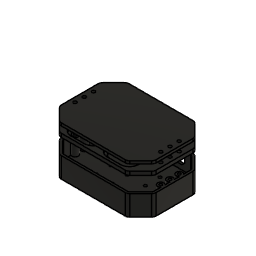
main (Autodesk Fusion 360 design; units mm, degrees)
Autodesk Fusion 360 part; units mm, degrees
sketch "main" plane through (0, 0, 16) normal (0, 0, 1) x (-1, 0, 0)
  line L0 (-15.9568, -31.9728) -> (-28.9568, -28.4593)
  arc A0 (-34.5, -21.219) -> (-28.9568, -28.4593) centre (-27, -21.219) ccw
  line L1 (-34.5, -21.219) -> (-34.5, 21.219)
  arc A1 (-28.9568, 28.4593) -> (-34.5, 21.219) centre (-27, 21.219) ccw
  line L2 (-28.9568, 28.4593) -> (-15.9568, 31.9728)
  arc A2 (-6.5, 24.7326) -> (-15.9568, 31.9728) centre (-14, 24.7326) ccw
  line L3 (-6.5, 24.7326) -> (-6.5, -24.7326)
  arc A3 (-15.9568, -31.9728) -> (-6.5, -24.7326) centre (-14, -24.7326) ccw
  line L4 (-7.8009, -43.5) -> (0, -43.5)
  line L5 (0, -43.5) -> (7.8009, -43.5)
  line L6 (7.8009, -43.5) -> (40.1741, -34.7505)
  arc A4 (40.1741, -34.7505) -> (43.5, -30.4063) centre (39, -30.4063) ccw
  line L7 (43.5, -30.4063) -> (43.5, 30.4063)
  arc A5 (43.5, 30.4063) -> (40.1741, 34.7505) centre (39, 30.4063) ccw
  line L8 (40.1741, 34.7505) -> (7.8009, 43.5)
  line L9 (7.8009, 43.5) -> (-7.8009, 43.5)
  line L10 (-7.8009, 43.5) -> (-40.1741, 34.7505)
  arc A6 (-40.1741, 34.7505) -> (-43.5, 30.4063) centre (-39, 30.4063) ccw
  line L11 (-43.5, 30.4063) -> (-43.5, -30.4063)
  arc A7 (-43.5, -30.4063) -> (-40.1741, -34.7505) centre (-39, -30.4063) ccw
  line L12 (-40.1741, -34.7505) -> (-7.8009, -43.5)
  arc A8 (6.5, -24.7326) -> (15.9568, -31.9728) centre (14, -24.7326) ccw
  line L13 (6.5, -24.7326) -> (6.5, 24.7326)
  arc A9 (15.9568, 31.9728) -> (6.5, 24.7326) centre (14, 24.7326) ccw
  line L14 (15.9568, 31.9728) -> (28.9568, 28.4593)
  arc A10 (34.5, 21.219) -> (28.9568, 28.4593) centre (27, 21.219) ccw
  line L15 (34.5, 21.219) -> (34.5, -21.219)
  arc A11 (28.9568, -28.4593) -> (34.5, -21.219) centre (27, -21.219) ccw
  line L16 (28.9568, -28.4593) -> (15.9568, -31.9728)
  line L17 (37, 34.5) -> (-37, 34.5) construction
  line L18 (-37, 34.5) -> (-37, -34.5) construction
  line L19 (-37, -34.5) -> (37, -34.5) construction
  line L20 (37, -34.5) -> (37, 34.5) construction
  line L21 (37, 34.5) -> (-37, -34.5) construction
  line L22 (-37, 34.5) -> (37, -34.5) construction
  line L23 (-37, -34.5) -> (-3, -34.5) construction
  line L24 (-3, -34.5) -> (-3, -0.5) construction
  line L25 (-3, -0.5) -> (-37, -0.5) construction
  line L26 (-37, -0.5) -> (-37, -34.5) construction
  line L27 (-37, 34.5) -> (-3, 34.5) construction
  line L28 (-3, 34.5) -> (-3, 0.5) construction
  line L29 (-3, 0.5) -> (-37, 0.5) construction
  line L30 (-37, 0.5) -> (-37, 34.5) construction
  line L31 (37, 34.5) -> (3, 34.5) construction
  line L32 (3, 34.5) -> (3, 0.5) construction
  line L33 (3, 0.5) -> (37, 0.5) construction
  line L34 (37, 0.5) -> (37, 34.5) construction
  line L35 (37, -34.5) -> (3, -34.5) construction
  line L36 (3, -34.5) -> (3, -0.5) construction
  line L37 (3, -0.5) -> (37, -0.5) construction
  line L38 (37, -0.5) -> (37, -34.5) construction
  line L39 (-37, -0.5) -> (-3, -34.5) construction
  line L40 (-3, -0.5) -> (-37, -34.5) construction
  line L41 (-37, 34.5) -> (-3, 0.5) construction
  line L42 (-3, 34.5) -> (-37, 0.5) construction
  line L43 (3, 34.5) -> (37, 0.5) construction
  line L44 (37, 34.5) -> (3, 0.5) construction
  line L45 (3, -34.5) -> (37, -0.5) construction
  line L46 (37, -34.5) -> (3, -0.5) construction
  line L47 (-12.7, -0.2) -> (-27.3, -0.2)
  line L48 (-37.3, -10.2) -> (-37.3, -24.8)
  line L49 (-27.3, -34.8) -> (-12.7, -34.8)
  line L50 (-2.7, -24.8) -> (-2.7, -10.2)
  line L51 (-2.7, -0.2) -> (-37.3, -34.8) construction
  line L52 (-37.3, -0.2) -> (-2.7, -34.8) construction
  line L53 (-12.7, 34.8) -> (-27.3, 34.8)
  line L54 (-37.3, 24.8) -> (-37.3, 10.2)
  line L55 (-27.3, 0.2) -> (-12.7, 0.2)
  line L56 (-2.7, 10.2) -> (-2.7, 24.8)
  line L57 (-2.7, 34.8) -> (-37.3, 0.2) construction
  line L58 (-37.3, 34.8) -> (-2.7, 0.2) construction
  line L59 (27.3, 34.8) -> (12.7, 34.8)
  line L60 (2.7, 24.8) -> (2.7, 10.2)
  line L61 (12.7, 0.2) -> (27.3, 0.2)
  line L62 (37.3, 10.2) -> (37.3, 24.8)
  line L63 (37.3, 34.8) -> (2.7, 0.2) construction
  line L64 (2.7, 34.8) -> (37.3, 0.2) construction
  line L65 (27.3, -0.2) -> (12.7, -0.2)
  line L66 (2.7, -10.2) -> (2.7, -24.8)
  line L67 (12.7, -34.8) -> (27.3, -34.8)
  line L68 (37.3, -24.8) -> (37.3, -10.2)
  line L69 (37.3, -0.2) -> (2.7, -34.8) construction
  line L70 (2.7, -0.2) -> (37.3, -34.8) construction
  arc A12 (-27.3, 34.8) -> (-37.3, 24.8) centre (-27.3, 24.8) ccw
  arc A13 (-37.3, 10.2) -> (-27.3, 0.2) centre (-27.3, 10.2) ccw
  arc A14 (-12.7, 0.2) -> (-2.7, 10.2) centre (-12.7, 10.2) ccw
  arc A15 (-2.7, 24.8) -> (-12.7, 34.8) centre (-12.7, 24.8) ccw
  arc A16 (12.7, 34.8) -> (2.7, 24.8) centre (12.7, 24.8) ccw
  arc A17 (37.3, 24.8) -> (27.3, 34.8) centre (27.3, 24.8) ccw
  arc A18 (27.3, 0.2) -> (37.3, 10.2) centre (27.3, 10.2) ccw
  arc A19 (2.7, 10.2) -> (12.7, 0.2) centre (12.7, 10.2) ccw
  arc A20 (-37.3, -24.8) -> (-27.3, -34.8) centre (-27.3, -24.8) ccw
  arc A21 (-12.7, -34.8) -> (-2.7, -24.8) centre (-12.7, -24.8) ccw
  arc A22 (-2.7, -10.2) -> (-12.7, -0.2) centre (-12.7, -10.2) ccw
  arc A23 (-27.3, -0.2) -> (-37.3, -10.2) centre (-27.3, -10.2) ccw
  arc A24 (12.7, -0.2) -> (2.7, -10.2) centre (12.7, -10.2) ccw
  arc A25 (2.7, -24.8) -> (12.7, -34.8) centre (12.7, -24.8) ccw
  arc A26 (27.3, -34.8) -> (37.3, -24.8) centre (27.3, -24.8) ccw
  arc A27 (37.3, -10.2) -> (27.3, -0.2) centre (27.3, -10.2) ccw
  arc A28 (-34.3, -24.8) -> (-27.3, -31.8) centre (-27.3, -24.8) ccw
  line L71 (-27.3, -31.8) -> (-12.7, -31.8)
  arc A29 (-12.7, -31.8) -> (-5.7, -24.8) centre (-12.7, -24.8) ccw
  line L72 (-5.7, -24.8) -> (-5.7, -10.2)
  arc A30 (-5.7, -10.2) -> (-12.7, -3.2) centre (-12.7, -10.2) ccw
  line L73 (-12.7, -3.2) -> (-27.3, -3.2)
  arc A31 (-27.3, -3.2) -> (-34.3, -10.2) centre (-27.3, -10.2) ccw
  line L74 (-34.3, -10.2) -> (-34.3, -24.8)
  arc A32 (-12.7, 3.2) -> (-5.7, 10.2) centre (-12.7, 10.2) ccw
  line L75 (-5.7, 10.2) -> (-5.7, 24.8)
  arc A33 (-5.7, 24.8) -> (-12.7, 31.8) centre (-12.7, 24.8) ccw
  line L76 (-12.7, 31.8) -> (-27.3, 31.8)
  arc A34 (-27.3, 31.8) -> (-34.3, 24.8) centre (-27.3, 24.8) ccw
  line L77 (-34.3, 24.8) -> (-34.3, 10.2)
  arc A35 (-34.3, 10.2) -> (-27.3, 3.2) centre (-27.3, 10.2) ccw
  line L78 (-27.3, 3.2) -> (-12.7, 3.2)
  line L79 (5.7, 24.8) -> (5.7, 10.2)
  arc A36 (5.7, 10.2) -> (12.7, 3.2) centre (12.7, 10.2) ccw
  line L80 (12.7, 3.2) -> (27.3, 3.2)
  arc A37 (27.3, 3.2) -> (34.3, 10.2) centre (27.3, 10.2) ccw
  line L81 (34.3, 10.2) -> (34.3, 24.8)
  arc A38 (34.3, 24.8) -> (27.3, 31.8) centre (27.3, 24.8) ccw
  line L82 (27.3, 31.8) -> (12.7, 31.8)
  arc A39 (12.7, 31.8) -> (5.7, 24.8) centre (12.7, 24.8) ccw
  arc A40 (12.7, -3.2) -> (5.7, -10.2) centre (12.7, -10.2) ccw
  line L83 (5.7, -10.2) -> (5.7, -24.8)
  arc A41 (5.7, -24.8) -> (12.7, -31.8) centre (12.7, -24.8) ccw
  line L84 (12.7, -31.8) -> (27.3, -31.8)
  arc A42 (27.3, -31.8) -> (34.3, -24.8) centre (27.3, -24.8) ccw
  line L85 (34.3, -24.8) -> (34.3, -10.2)
  arc A43 (34.3, -10.2) -> (27.3, -3.2) centre (27.3, -10.2) ccw
  line L86 (27.3, -3.2) -> (12.7, -3.2)
  line L87 (35.4289, 37.5) -> (-35.4289, 37.5)
  line L88 (-52.5, 20.4289) -> (-52.5, -20.4289)
  line L89 (-35.4289, -37.5) -> (35.4289, -37.5)
  line L90 (52.5, -20.4289) -> (52.5, 20.4289)
  line L91 (52.5, 37.5) -> (-52.5, -37.5) construction
  line L92 (-52.5, 37.5) -> (52.5, -37.5) construction
  line L93 (-38.9645, -36.0355) -> (-51.0355, -23.9645)
  line L94 (-38.9645, 36.0355) -> (-51.0355, 23.9645)
  line L95 (38.9645, 36.0355) -> (51.0355, 23.9645)
  line L96 (38.9645, -36.0355) -> (51.0355, -23.9645)
  arc A44 (-38.9645, -36.0355) -> (-35.4289, -37.5) centre (-35.4289, -32.5) ccw
  arc A45 (-52.5, -20.4289) -> (-51.0355, -23.9645) centre (-47.5, -20.4289) ccw
  arc A46 (-51.0355, 23.9645) -> (-52.5, 20.4289) centre (-47.5, 20.4289) ccw
  arc A47 (-35.4289, 37.5) -> (-38.9645, 36.0355) centre (-35.4289, 32.5) ccw
  arc A48 (38.9645, 36.0355) -> (35.4289, 37.5) centre (35.4289, 32.5) ccw
  arc A49 (52.5, 20.4289) -> (51.0355, 23.9645) centre (47.5, 20.4289) ccw
  arc A50 (51.0355, -23.9645) -> (52.5, -20.4289) centre (47.5, -20.4289) ccw
  arc A51 (35.4289, -37.5) -> (38.9645, -36.0355) centre (35.4289, -32.5) ccw
  line L97 (-52.5, 20.4289) -> (-42.5, 20.4289) construction
  line L98 (-42.5, 20.4289) -> (-42.5, -20.4289) construction
  line L99 (-42.5, -20.4289) -> (-52.5, -20.4289) construction
  line L100 (-52.5, -20.4289) -> (-52.5, 20.4289) construction
  line L101 (-52.5, 20.4289) -> (-42.5, -20.4289) construction
  line L102 (-42.5, 20.4289) -> (-52.5, -20.4289) construction
  circle A52 centre (-47.5, 0) radius 1.8
  line L103 (-52.5, 20.4289) -> (-42.5, 0) construction
  line L104 (-42.5, 20.4289) -> (-52.5, 0) construction
  line L105 (-52.5, -20.4289) -> (-42.5, 0) construction
  line L106 (-42.5, -20.4289) -> (-52.5, 0) construction
  circle A53 centre (-47.5, -10.2145) radius 1.8
  circle A54 centre (-47.5, 10.2145) radius 1.8
  line L107 (52.5, 20.4289) -> (52.5, -20.4289)
  line L108 (52.5, 20.4289) -> (42.5, 20.4289) construction
  line L109 (42.5, 20.4289) -> (42.5, -20.4291) construction
  line L110 (42.5, -20.4291) -> (52.5, -20.4291) construction
  line L111 (52.5, -20.4291) -> (52.5, 20.4289) construction
  line L112 (42.5, 20.4289) -> (52.5, -20.4289) construction
  line L113 (52.5, 20.4289) -> (42.5, -20.4291) construction
  line L114 (42.5, 20.4289) -> (52.5, 0) construction
  line L115 (52.5, 20.4289) -> (42.5, -0.0001) construction
  line L116 (42.5, -0.0001) -> (52.5, -20.4289) construction
  line L117 (52.5, 0) -> (42.5, -20.4291) construction
  circle A55 centre (47.5, 10.2145) radius 1.8
  circle A56 centre (47.5, -0.0001) radius 1.8
  circle A57 centre (47.5, -10.2145) radius 1.8
  point P0 (-20, -17.5)
  point P1 (-20, 17.5)
  point P2 (20, 17.5)
  point P3 (20, -17.5)
  point P4 (-37.5, -37.5)
  point P5 (-52.5, -22.5)
  point P6 (-37.5, 37.5)
  point P7 (-52.5, 22.5)
  point P8 (37.5, 37.5)
  point P9 (52.5, 22.5)
  point P10 (37.5, -37.5)
  point P11 (52.5, -22.5)
  dimension "d3" = 74
  dimension "d4" = 69
  dimension "d5" = 34
  dimension "d6" = 34
  dimension "d7" = 34
  dimension "d8" = 34
  dimension "d9" = 34
  dimension "d10" = 34
  dimension "d11" = 34
  dimension "d12" = 34
  dimension "d13" = 34.6
  dimension "d14" = 34.6
  dimension "d15" = 34.6
  dimension "d16" = 34.6
  dimension "d17" = 34.6
  dimension "d18" = 34.6
  dimension "d19" = 34.6
  dimension "d20" = 34.6
  dimension "d21" = 10
  dimension "d22" = 10
  dimension "d23" = 10
  dimension "d24" = 10
  dimension "d25" = 10
  dimension "d26" = 10
  dimension "d27" = 10
  dimension "d28" = 10
  dimension "d29" = 10
  dimension "d30" = 10
  dimension "d31" = 10
  dimension "d32" = 10
  dimension "d33" = 10
  dimension "d34" = 10
  dimension "d35" = 10
  dimension "d36" = 10
  dimension "d37" = -3
  dimension "d38" = -3
  dimension "d39" = -3
  dimension "d40" = -3
  dimension "d41" = 105
  dimension "d42" = 75
  dimension "d43" = 15
  dimension "d44" = 15
  dimension "d45" = 15
  dimension "d46" = 15
  dimension "d47" = 15
  dimension "d48" = 15
  dimension "d49" = 15
  dimension "d50" = 15
  dimension "d51" = 5
  dimension "d52" = 5
  dimension "d53" = 5
  dimension "d54" = 5
  dimension "d55" = 5
  dimension "d56" = 5
  dimension "d57" = 5
  dimension "d58" = 5
  dimension "d70" = 10
  dimension "d72" = 3.6
  dimension "d74" = 3.6
  dimension "d75" = 3.6
  dimension "d80" = 10
  dimension "d81" = 40.858
  dimension "d82" = 3.6
  dimension "d83" = 3.6
  dimension "d84" = 3.6
  constraint horizontal L17
  constraint perpendicular L17 L18
  constraint parallel L17 L19
  constraint parallel L18 L20
  constraint coincident L21 origin
  constraint coincident L22 origin
  constraint horizontal L23
  constraint vertical L24
  constraint horizontal L25
  constraint vertical L26
  constraint horizontal L27
  constraint vertical L28
  constraint horizontal L29
  constraint vertical L30
  constraint horizontal L31
  constraint vertical L32
  constraint horizontal L33
  constraint vertical L34
  constraint horizontal L35
  constraint vertical L36
  constraint horizontal L37
  constraint vertical L38
  constraint horizontal L47
  constraint perpendicular L47 L48
  constraint parallel L47 L49
  constraint parallel L48 L50
  constraint coincident L51 P0
  constraint coincident L52 P0
  constraint midpoint L39 P0
  constraint horizontal L53
  constraint perpendicular L53 L54
  constraint parallel L53 L55
  constraint parallel L54 L56
  constraint coincident L57 P1
  constraint coincident L58 P1
  constraint midpoint L42 P1
  constraint horizontal L59
  constraint perpendicular L59 L60
  constraint parallel L59 L61
  constraint parallel L60 L62
  constraint coincident L63 P2
  constraint coincident L64 P2
  constraint midpoint L44 P2
  constraint horizontal L65
  constraint perpendicular L65 L66
  constraint parallel L65 L67
  constraint parallel L66 L68
  constraint coincident L69 P3
  constraint coincident L70 P3
  constraint midpoint L46 P3
  constraint coincident L58.start L54
  constraint coincident L58.start L53
  constraint tangent L54 A12
  constraint tangent L53 A12
  constraint coincident L57.end L55
  constraint coincident L57.end L54
  constraint tangent L55 A13
  constraint tangent L54 A13
  constraint coincident L58.end L55
  constraint coincident L58.end L56
  constraint tangent L55 A14
  constraint tangent L56 A14
  constraint coincident L57.start L56
  constraint coincident L57.start L53
  constraint tangent L56 A15
  constraint tangent L53 A15
  constraint coincident L64.start L59
  constraint coincident L64.start L60
  constraint tangent L59 A16
  constraint tangent L60 A16
  constraint coincident L63.start L59
  constraint coincident L63.start L62
  constraint tangent L59 A17
  constraint tangent L62 A17
  constraint coincident L64.end L62
  constraint coincident L64.end L61
  constraint tangent L62 A18
  constraint tangent L61 A18
  constraint coincident L63.end L61
  constraint coincident L63.end L60
  constraint tangent L61 A19
  constraint tangent L60 A19
  constraint coincident L51.end L49
  constraint coincident L51.end L48
  constraint tangent L49 A20
  constraint tangent L48 A20
  constraint coincident L52.end L49
  constraint coincident L52.end L50
  constraint tangent L49 A21
  constraint tangent L50 A21
  constraint coincident L51.start L50
  constraint coincident L51.start L47
  constraint tangent L50 A22
  constraint tangent L47 A22
  constraint coincident L52.start L47
  constraint coincident L52.start L48
  constraint tangent L47 A23
  constraint tangent L48 A23
  constraint coincident L70.start L66
  constraint coincident L70.start L65
  constraint tangent L66 A24
  constraint tangent L65 A24
  constraint coincident L69.end L67
  constraint coincident L69.end L66
  constraint tangent L67 A25
  constraint tangent L66 A25
  constraint coincident L70.end L67
  constraint coincident L70.end L68
  constraint tangent L67 A26
  constraint tangent L68 A26
  constraint coincident L69.start L68
  constraint coincident L69.start L65
  constraint tangent L68 A27
  constraint tangent L65 A27
  constraint horizontal L87
  constraint perpendicular L87 L88
  constraint parallel L87 L89
  constraint parallel L88 L90
  constraint coincident L91 origin
  constraint coincident L92 origin
  constraint coincident L91.end L89
  constraint coincident L91.end L88
  constraint coincident L92.start L87
  constraint coincident L92.start L88
  constraint coincident L91.start L87
  constraint coincident L91.start L90
  constraint coincident L92.end L89
  constraint coincident L92.end L90
  constraint coincident L89 P4
  constraint coincident P4 L93
  constraint tangent L89 A44
  constraint tangent L93 A44
  constraint coincident P5 L93
  constraint coincident L88 P5
  constraint tangent L93 A45
  constraint tangent L88 A45
  constraint coincident P7 L94
  constraint coincident L88 P7
  constraint tangent L94 A46
  constraint tangent L88 A46
  constraint coincident P6 L94
  constraint coincident L87 P6
  constraint tangent L94 A47
  constraint tangent L87 A47
  constraint coincident P8 L95
  constraint coincident L87 P8
  constraint tangent L95 A48
  constraint tangent L87 A48
  constraint coincident P9 L95
  constraint coincident L90 P9
  constraint tangent L95 A49
  constraint tangent L90 A49
  constraint coincident P11 L96
  constraint coincident L90 P11
  constraint tangent L96 A50
  constraint tangent L90 A50
  constraint coincident P10 L96
  constraint coincident L89 P10
  constraint tangent L96 A51
  constraint tangent L89 A51
  constraint horizontal L97
  constraint vertical L98
  constraint horizontal L99
  constraint vertical L100
  constraint midpoint L101 A52.centre
  constraint midpoint L98 L103.end
  constraint midpoint L100 L104.end
  constraint midpoint L106 A53.centre
  constraint midpoint L104 A54.centre
  constraint horizontal L108
  constraint vertical L109
  constraint horizontal L110
  constraint vertical L111
  constraint midpoint L107 L114.end
  constraint midpoint L109 L115.end
  constraint midpoint L114 A55.centre
  constraint midpoint L113 A56.centre
  constraint midpoint L117 A57.centre
  measures "d3" distance of L18.end L19.end
  measures "d4" distance of L17.end L18.end
  measures "d5" distance of L18.end L23.end
  measures "d6" distance of L18.end L25.end
  measures "d7" distance of L17.end L27.end
  measures "d8" distance of L17.end L29.end
  measures "d9" distance of L17.start L31.end
  measures "d10" distance of L17.start L33.end
  measures "d11" distance of L19.end L35.end
  measures "d12" distance of L19.end L37.end
  measures "d13" distance of L51.end L52.end
  measures "d14" distance of L52.start L51.end
  measures "d15" distance of L57.end L58.end
  measures "d16" distance of L58.start L57.end
  measures "d17" distance of L63.end L64.end
  measures "d18" distance of L64.start L63.end
  measures "d19" distance of L69.end L70.end
  measures "d20" distance of L70.start L69.end
  measures "d21" radius of A12
  measures "d22" radius of A13
  measures "d23" radius of A14
  measures "d24" radius of A15
  measures "d25" radius of A16
  measures "d26" radius of A17
  measures "d27" radius of A18
  measures "d28" radius of A19
  measures "d29" radius of A20
  measures "d30" radius of A21
  measures "d31" radius of A22
  measures "d32" radius of A23
  measures "d33" radius of A24
  measures "d34" radius of A25
  measures "d35" radius of A26
  measures "d36" radius of A27
  measures "d41" distance of L91.end L92.end
  measures "d42" distance of L92.start L91.end
  measures "d43" distance of L91.end P4
  measures "d44" distance of L91.end P5
  measures "d45" distance of L92.start P6
  measures "d46" distance of L92.start P7
  measures "d47" distance of L91.start P8
  measures "d48" distance of L91.start P9
  measures "d49" distance of L92.end P10
  measures "d50" distance of L92.end P11
  measures "d51" radius of A44
  measures "d52" radius of A45
  measures "d53" radius of A46
  measures "d54" radius of A47
  measures "d55" radius of A48
  measures "d56" radius of A49
  measures "d57" radius of A50
  measures "d58" radius of A51
  measures "d70" distance of L88.start L97.end
  measures "d72" diameter of A52
  measures "d74" diameter of A53
  measures "d75" diameter of A54
  measures "d80" distance of L90.end L108.end
  measures "d81" distance of L90.end L110.end
  measures "d82" diameter of A55
  measures "d83" diameter of A56
  measures "d84" diameter of A57
extrude "Extrude1" add sketch "main" along normal blind 1 contours L0 A0 L1 L3 A3 L48 L49 L50 A20 A21 A22 A23 A28 L71 A29 L72 A30 L74 | L0 A3 L71 A29 | A0 L1 L3 L47 A22 A23 A30 L73 A31 L74 | L1 L3 L47 L55 A13 A14 A22 A23 | L1 A1 L3 L55 A13 A14 A32 L77 A35 L78 | L1 A1 L2 A2 L3 L53 L54 L56 A12 A13 A14 A15 A32 L75 A33 L76 A34 L77 | L2 A2 A33 L76 | A7 L12 L89 L93 A44 | L6 A4 L7 A5 L8 L10 A6 L11 A7 L12 L87 L89 L93 L94 L95 L96 | L6 A4 L89 L96 A51 | A6 L11 A7 L88 L93 L94 A45 A46 | A4 L7 A5 L90 L95 L96 A49 A50 L107 | L10 A6 L87 L94 A47 | A5 L8 L87 L95 A48 | A8 L16 A41 L84 | A8 L13 L15 A11 L16 L66 L67 L68 A24 A25 A26 A27 A40 L83 A41 L84 A42 L85 | L13 L15 A11 L65 A24 A27 A40 L85 A43 L86 | L13 L15 L61 L65 A18 A19 A24 A27 | L13 A9 L14 A10 L15 L59 L60 L62 A16 A17 A18 A19 L79 A36 L81 A38 L82 A39 | L13 A10 L15 L61 A18 A19 A36 L80 A37 L81 | A9 L14 L82 A39 | A52 | A53 | A54 | A55 | A56 | A57 makes body 1
extrude "Extrude2" add sketch "main" along normal blind 3 from surface at 1 contours L1 L3 L47 L55 A13 A14 A22 A23 | A7 L12 L89 L93 A44 | L6 A4 L7 A5 L8 L10 A6 L11 A7 L12 L87 L89 L93 L94 L95 L96 | L6 A4 L89 L96 A51 | A6 L11 A7 L88 L93 L94 A45 A46 | A4 L7 A5 L90 L95 L96 A49 A50 L107 | L10 A6 L87 L94 A47 | A5 L8 L87 L95 A48 | L13 L15 L61 L65 A18 A19 A24 A27 | A52 | A53 | A54 | A55 | A56 | A57 bodies 1
extrude "Extrude3" add sketch "main" along normal blind 3 from surface at 11 separate body contours L0 A0 L1 L3 A3 L48 L49 L50 A20 A21 A22 A23 A28 L71 A29 L72 A30 L74 | L0 A3 L71 A29 | L0 A0 A28 L71 L74 | L0 A0 L3 A3 L71 A29 A30 L73 A31 L74 | L3 A3 A29 L72 A30 | A0 L1 L3 L47 A22 A23 A30 L73 A31 L74 | L1 L3 L47 L55 A13 A14 A22 A23 | L1 A1 L3 L55 A13 A14 A32 L77 A35 L78 | L1 A1 L2 A2 L3 L53 L54 L56 A12 A13 A14 A15 A32 L75 A33 L76 A34 L77 | A1 L2 A2 L3 A32 A33 L76 L77 A35 L78 | A2 L3 A32 L75 A33 | A1 L2 L76 A34 L77 | L2 A2 A33 L76 | A7 L12 L89 L93 A44 | L6 A4 L7 A5 L8 L10 A6 L11 A7 L12 L87 L89 L93 L94 L95 L96 | L6 A4 L89 L96 A51 | A6 L11 A7 L88 L93 L94 A45 A46 | A4 L7 A5 L90 L95 L96 A49 A50 L107 | L10 A6 L87 L94 A47 | A5 L8 L87 L95 A48 | A8 L13 A11 L16 A40 A41 L84 L85 A43 L86 | A8 L13 A40 L83 A41 | A8 L16 A41 L84 | A8 L13 L15 A11 L16 L66 L67 L68 A24 A25 A26 A27 A40 L83 A41 L84 A42 L85 | L13 L15 A11 L65 A24 A27 A40 L85 A43 L86 | L13 L15 L61 L65 A18 A19 A24 A27 | A11 L16 L84 A42 L85 | L13 A9 L14 A10 L15 L59 L60 L62 A16 A17 A18 A19 L79 A36 L81 A38 L82 A39 | L13 A10 L15 L61 A18 A19 A36 L80 A37 L81 | L13 A9 L79 A36 A39 | L13 A9 L14 A10 A36 L80 A37 L81 L82 A39 | A9 L14 L82 A39 | L14 A10 L81 A38 L82 | A52 | A53 | A54 | A55 | A56 | A57 makes body 2
extrude "Extrude4" add sketch "main" against normal blind 1.5 from surface at 11 contours L0 A0 A28 L71 L74 | L0 A0 L3 A3 L71 A29 A30 L73 A31 L74 | L3 A3 A29 L72 A30 | A1 L2 A2 L3 A32 A33 L76 L77 A35 L78 | A2 L3 A32 L75 A33 | A1 L2 L76 A34 L77 | A8 L13 A11 L16 A40 A41 L84 L85 A43 L86 | A8 L13 A40 L83 A41 | A11 L16 L84 A42 L85 | L13 A9 L79 A36 A39 | L13 A9 L14 A10 A36 L80 A37 L81 L82 A39 | L14 A10 L81 A38 L82 bodies 2
extrude "Extrude5" cut sketch "main" along normal blind 14 contours A52 | A53 | A54 | A55 | A56 | A57 bodies 1 2
extrude "Extrude6" add sketch "main" against normal blind 24 from surface at -16 separate body contours L0 A0 L1 L3 A3 L48 L49 L50 A20 A21 A22 A23 A28 L71 A29 L72 A30 L74 | L0 A3 L71 A29 | L0 A0 A28 L71 L74 | L0 A0 L3 A3 L71 A29 A30 L73 A31 L74 | L3 A3 A29 L72 A30 | A0 L1 L3 L47 A22 A23 A30 L73 A31 L74 | L1 L3 L47 L55 A13 A14 A22 A23 | L1 A1 L3 L55 A13 A14 A32 L77 A35 L78 | L1 A1 L2 A2 L3 L53 L54 L56 A12 A13 A14 A15 A32 L75 A33 L76 A34 L77 | A1 L2 A2 L3 A32 A33 L76 L77 A35 L78 | A2 L3 A32 L75 A33 | A1 L2 L76 A34 L77 | L2 A2 A33 L76 | A7 L12 L89 L93 A44 | L6 A4 L7 A5 L8 L10 A6 L11 A7 L12 L87 L89 L93 L94 L95 L96 | L6 A4 L89 L96 A51 | A6 L11 A7 L88 L93 L94 A45 A46 | A4 L7 A5 L90 L95 L96 A49 A50 L107 | L10 A6 L87 L94 A47 | A5 L8 L87 L95 A48 | A8 L13 A11 L16 A40 A41 L84 L85 A43 L86 | A8 L13 A40 L83 A41 | A8 L16 A41 L84 | A8 L13 L15 A11 L16 L66 L67 L68 A24 A25 A26 A27 A40 L83 A41 L84 A42 L85 | L13 L15 A11 L65 A24 A27 A40 L85 A43 L86 | L13 L15 L61 L65 A18 A19 A24 A27 | A11 L16 L84 A42 L85 | L13 A9 L14 A10 L15 L59 L60 L62 A16 A17 A18 A19 L79 A36 L81 A38 L82 A39 | L13 A10 L15 L61 A18 A19 A36 L80 A37 L81 | L13 A9 L79 A36 A39 | L13 A9 L14 A10 A36 L80 A37 L81 L82 A39 | A9 L14 L82 A39 | L14 A10 L81 A38 L82 | A52 | A53 | A54 | A55 | A56 | A57 makes body 3
sketch "mounting-screws" plane through (0, 0, 0) normal (0, 0, 1) x (-1, 0, 0)
  arc A0 (38.9645, 36.0355) -> (35.4289, 37.5) centre (35.4289, 32.5) ccw
  line L0 (35.4289, 37.5) -> (-35.4289, 37.5)
  arc A1 (-35.4289, 37.5) -> (-38.9645, 36.0355) centre (-35.4289, 32.5) ccw
  line L1 (-38.9645, 36.0355) -> (-51.0355, 23.9645)
  arc A2 (-51.0355, 23.9645) -> (-52.5, 20.4289) centre (-47.5, 20.4289) ccw
  line L2 (-52.5, 20.4289) -> (-52.5, -20.4289)
  arc A3 (-52.5, -20.4289) -> (-51.0355, -23.9645) centre (-47.5, -20.4289) ccw
  line L3 (-51.0355, -23.9645) -> (-38.9645, -36.0355)
  arc A4 (-38.9645, -36.0355) -> (-35.4289, -37.5) centre (-35.4289, -32.5) ccw
  line L4 (-35.4289, -37.5) -> (35.4289, -37.5)
  arc A5 (35.4289, -37.5) -> (38.9645, -36.0355) centre (35.4289, -32.5) ccw
  line L5 (38.9645, -36.0355) -> (51.0355, -23.9645)
  arc A6 (51.0355, -23.9645) -> (52.5, -20.4289) centre (47.5, -20.4289) ccw
  line L6 (52.5, -20.4289) -> (52.5, 20.4289)
  arc A7 (52.5, 20.4289) -> (51.0355, 23.9645) centre (47.5, 20.4289) ccw
  line L7 (51.0355, 23.9645) -> (38.9645, 36.0355)
  line L8 (37.1967, -34.2678) -> (49.2678, -22.1967)
  arc A8 (49.2678, -22.1967) -> (50, -20.4289) centre (47.5, -20.4289) ccw
  line L9 (50, -20.4289) -> (50, 20.4289)
  arc A9 (50, 20.4289) -> (49.2678, 22.1967) centre (47.5, 20.4289) ccw
  line L10 (49.2678, 22.1967) -> (37.1967, 34.2678)
  arc A10 (37.1967, 34.2678) -> (35.4289, 35) centre (35.4289, 32.5) ccw
  line L11 (35.4289, 35) -> (-35.4289, 35)
  arc A11 (-35.4289, 35) -> (-37.1967, 34.2678) centre (-35.4289, 32.5) ccw
  line L12 (-37.1967, 34.2678) -> (-49.2678, 22.1967)
  arc A12 (-49.2678, 22.1967) -> (-50, 20.4289) centre (-47.5, 20.4289) ccw
  line L13 (-50, 20.4289) -> (-50, -20.4289)
  arc A13 (-50, -20.4289) -> (-49.2678, -22.1967) centre (-47.5, -20.4289) ccw
  line L14 (-49.2678, -22.1967) -> (-37.1967, -34.2678)
  arc A14 (-37.1967, -34.2678) -> (-35.4289, -35) centre (-35.4289, -32.5) ccw
  line L15 (-35.4289, -35) -> (35.4289, -35)
  arc A15 (35.4289, -35) -> (37.1967, -34.2678) centre (35.4289, -32.5) ccw
  circle A16 centre (47.5, -10.2145) radius 1.55
  circle A17 centre (47.5, 10.2145) radius 1.55
  circle A18 centre (47.5, -0.0001) radius 1.55
  circle A19 centre (-47.5, -10.2145) radius 1.55
  circle A20 centre (-47.5, 0) radius 1.55
  circle A21 centre (-47.5, 10.2145) radius 1.55
  circle A22 centre (47.5, 10.2145) radius 3.5
  circle A23 centre (47.5, -0.0001) radius 3.5
  circle A24 centre (47.5, -10.2145) radius 3.5
  circle A25 centre (-47.5, -10.2145) radius 3.5
  circle A26 centre (-47.5, 0) radius 3.5
  circle A27 centre (-47.5, 10.2145) radius 3.5
  point P0 (47.5, -10.2145)
  point P1 (47.5, 10.2145)
  point P2 (47.5, -0.0001)
  point P3 (-47.5, -10.2145)
  point P4 (-47.5, 0)
  point P5 (-47.5, 10.2145)
  dimension "d88" = -2.5
  dimension "d91" = 3.1
  dimension "d92" = 3.1
  dimension "d93" = 3.1
  dimension "d94" = 3.1
  dimension "d95" = 3.1
  dimension "d96" = 3.1
  dimension "d97" = 7
  dimension "d98" = 7
  dimension "d99" = 7
  dimension "d100" = 7
  dimension "d101" = 7
  dimension "d102" = 7
  constraint coincident P0 A16.centre
  constraint coincident P1 A17.centre
  constraint coincident P2 A18.centre
  constraint coincident P3 A19.centre
  constraint coincident P4 A20.centre
  constraint coincident P5 A21.centre
  constraint concentric A19 A25
  constraint concentric A20 A26
  measures "d91" diameter of A16
  measures "d92" diameter of A17
  measures "d93" diameter of A18
  measures "d94" diameter of A19
  measures "d95" diameter of A20
  measures "d96" diameter of A21
  measures "d97" diameter of A22
  measures "d98" diameter of A23
  measures "d99" diameter of A24
  measures "d100" diameter of A25
  measures "d101" diameter of A26
  measures "d102" diameter of A27
extrude "Extrude7" cut sketch "mounting-screws" against normal blind 21 contours L8 A8 L9 A9 L10 A10 L11 A11 L12 A12 L13 A13 L14 A14 L15 A15 A22 A23 A24 A25 A26 A27 | L9 A24 | L9 A23 | L13 A25 | L9 A22 | L13 A26 | L13 A27 | A16 | A17 | A18 | A19 | A20 | A21 picked at (49.6833, -10.2145) picked at (49.6833, -0.0001) picked at (-49.6833, -10.2145) picked at (49.6833, 10.2145) picked at (-49.6833, 0) picked at (-49.6833, 10.2145) bodies 3
extrude "Extrude8" add sketch "mounting-screws" against normal blind 20 contours L9 A24 | L9 A23 | L13 A25 | L9 A22 | L13 A26 | L13 A27 picked at (49.6833, -10.2145) picked at (49.6833, -0.0001) picked at (-49.6833, -10.2145) picked at (49.6833, 10.2145) picked at (-49.6833, 0) picked at (-49.6833, 10.2145) bodies 3
sketch "electronics" plane through (0, 0, -21) normal (0, 0, 1) x (-1, 0, 0)
  line L0 (-50, 20.4289) -> (-50, -20.4289)
  arc A0 (-50, -20.4289) -> (-49.2678, -22.1967) centre (-47.5, -20.4289) ccw
  line L1 (-49.2678, -22.1967) -> (-37.1967, -34.2678)
  arc A1 (-37.1967, -34.2678) -> (-35.4289, -35) centre (-35.4289, -32.5) ccw
  line L2 (-35.4289, -35) -> (35.4289, -35)
  arc A2 (35.4289, -35) -> (37.1967, -34.2678) centre (35.4289, -32.5) ccw
  line L3 (37.1967, -34.2678) -> (49.2678, -22.1967)
  arc A3 (49.2678, -22.1967) -> (50, -20.4289) centre (47.5, -20.4289) ccw
  line L4 (50, -20.4289) -> (50, 20.4289)
  arc A4 (50, 20.4289) -> (49.2678, 22.1967) centre (47.5, 20.4289) ccw
  line L5 (49.2678, 22.1967) -> (37.1967, 34.2678)
  arc A5 (37.1967, 34.2678) -> (35.4289, 35) centre (35.4289, 32.5) ccw
  line L6 (35.4289, 35) -> (-35.4289, 35)
  arc A6 (-35.4289, 35) -> (-37.1967, 34.2678) centre (-35.4289, 32.5) ccw
  line L7 (-37.1967, 34.2678) -> (-49.2678, 22.1967)
  arc A7 (-49.2678, 22.1967) -> (-50, 20.4289) centre (-47.5, 20.4289) ccw
  line L8 (0, 35) -> (0, 25.1) construction
  line L9 (10.225, 17.2) -> (-10.225, 17.2)
  line L10 (-10.225, 17.2) -> (-10.225, 33)
  line L11 (-10.225, 33) -> (10.225, 33)
  line L12 (10.225, 33) -> (10.225, 17.2)
  line L13 (10.225, 17.2) -> (-10.225, 33) construction
  line L14 (-10.225, 17.2) -> (10.225, 33) construction
  line L15 (-12.225, 15.2) -> (-12.225, 35)
  line L16 (-12.225, 35) -> (12.225, 35)
  line L17 (12.225, 35) -> (12.225, 15.2)
  line L18 (12.225, 15.2) -> (-12.225, 15.2)
  line L19 (-12.225, 35) -> (-40.125, 35) construction
  line L20 (-40.125, 35) -> (-40.125, -35) construction
  line L21 (-40.125, -35) -> (-12.225, -35) construction
  line L22 (-12.225, -35) -> (-12.225, 35) construction
  line L23 (-12.225, 35) -> (-40.125, -35) construction
  line L24 (-12.225, -35) -> (-40.125, 35) construction
  line L25 (-12.225, -28) -> (-40.125, -28)
  line L26 (-40.125, -28) -> (-40.125, 28)
  line L27 (-40.125, 28) -> (-12.225, 28)
  line L28 (-12.225, 28) -> (-12.225, -28)
  line L29 (-12.225, -28) -> (-40.125, 28) construction
  line L30 (-40.125, -28) -> (-12.225, 28) construction
  line L31 (-42.125, -29) -> (-42.125, 29)
  line L32 (-41.125, 30) -> (-10.225, 30)
  line L33 (-10.225, 30) -> (-10.225, -30)
  line L34 (-10.225, -30) -> (-41.125, -30)
  line L35 (-42.125, 29) -> (-41.125, 30)
  line L36 (-41.125, -30) -> (-42.125, -29)
  line L37 (-26.175, 0) -> (-26.175, -30) construction
  line L38 (-26.175, -30) -> (-20.675, -30) construction
  line L39 (-20.675, -30) -> (-31.675, -30)
  line L40 (-31.675, -30) -> (-31.675, -28)
  line L41 (-31.675, -28) -> (-20.675, -28)
  line L42 (-20.675, -28) -> (-20.675, -30)
  line L43 (-10.225, 15.2) -> (10.225, 15.2)
  line L44 (10.225, 15.2) -> (10.225, -18.5)
  line L45 (10.225, -18.5) -> (-10.225, -18.5)
  line L46 (-10.225, -18.5) -> (-10.225, 15.2)
  line L47 (-12.225, -20.5) -> (-12.225, 17.2)
  line L48 (-12.225, 17.2) -> (12.225, 17.2)
  line L49 (12.225, 17.2) -> (12.225, -20.5)
  line L50 (12.225, -20.5) -> (-12.225, -20.5)
  line L51 (10.525, 16.9) -> (-10.525, 16.9)
  line L52 (-10.525, 16.9) -> (-10.525, 33.3)
  line L53 (-10.525, 33.3) -> (10.525, 33.3)
  line L54 (10.525, 33.3) -> (10.525, 16.9)
  line L55 (10.525, -18.8) -> (-10.525, -18.8)
  line L56 (-10.525, -18.8) -> (-10.525, 15.5)
  line L57 (-10.525, 15.5) -> (10.525, 15.5)
  line L58 (10.525, 15.5) -> (10.525, -18.8)
  line L59 (-11.925, -28.3) -> (-40.425, -28.3)
  line L60 (-40.425, -28.3) -> (-40.425, 28.3)
  line L61 (-40.425, 28.3) -> (-11.925, 28.3)
  line L62 (-11.925, 28.3) -> (-11.925, -28.3)
  circle A8 centre (7.8277, 30.2114) radius 1.5558
  line L63 (7.8277, 28.6556) -> (7.8277, 31.7671) construction
  circle A9 centre (7.8277, 30.2114) radius 1.5558
  circle A10 centre (-7.7298, 30.2114) radius 1.5558
  line L64 (-7.7298, 28.6556) -> (-7.7298, 31.7671) construction
  circle A11 centre (-7.7298, 30.2114) radius 1.5558
  point P0 (0, 25.1)
  point P1 (-26.175, 0)
  point P2 (-42.125, -30)
  point P3 (-42.125, 30)
  point P4 (7.8277, 28.6556)
  point P5 (-7.7298, 28.6556)
  dimension "d107" = 9.9
  dimension "d108" = 20.45
  dimension "d109" = 15.8
  dimension "d110" = -2
  dimension "d111" = 27.9
  dimension "d112" = 27.9
  dimension "d113" = 56
  dimension "d115" = 1
  dimension "d116" = 1
  dimension "d117" = 1
  dimension "d118" = 1
  dimension "d119" = 5.5
  dimension "d120" = 11
  dimension "d121" = 2
  dimension "d122" = 20.45
  dimension "d123" = 33.7
  dimension "d124" = -2
  dimension "d130" = -0.3
  dimension "d131" = -0.3
  dimension "d132" = -0.3
  constraint midpoint L6 L8.start
  constraint perpendicular L6 L8
  constraint horizontal L9
  constraint perpendicular L9 L10
  constraint parallel L9 L11
  constraint parallel L10 L12
  constraint coincident L13 P0
  constraint coincident L14 P0
  constraint coincident P0 L8.end
  constraint horizontal L19
  constraint vertical L20
  constraint horizontal L21
  constraint vertical L22
  constraint horizontal L25
  constraint perpendicular L25 L26
  constraint parallel L25 L27
  constraint parallel L26 L28
  constraint coincident L29 P1
  constraint coincident L30 P1
  constraint midpoint L23 P1
  constraint coincident P3 L31
  constraint coincident P3 L32
  constraint coincident P2 L34
  constraint coincident P2 L31
  constraint coincident P1 L37.start
  constraint coincident L34 L37.end
  constraint perpendicular L34 L37
  constraint perpendicular L37 L38
  constraint horizontal L39
  constraint vertical L40
  constraint horizontal L41
  constraint vertical L42
  constraint horizontal L43
  constraint vertical L44
  constraint horizontal L45
  constraint vertical L46
  constraint coincident L33 L43.start
  constraint coincident L18 L43.start
  constraint coincident P4 L63.start
  constraint coincident A8 L63.end
  constraint parallel L54 L63
  constraint concentric A8 A9
  constraint coincident P5 L64.start
  constraint coincident A10 L64.end
  constraint vertical L64
  constraint concentric A10 A11
  measures "d107" distance of L8.start P0
  measures "d108" distance of L10.end L11.end
  measures "d109" distance of L9.end L10.end
  measures "d111" distance of L15.end L19.end
  measures "d112" distance of L26.end L27.end
  measures "d113" distance of L25.end L26.end
  measures "d115" distance of P3 L31.end
  measures "d116" distance of P3 L32.start
  measures "d117" distance of P2 L34.end
  measures "d118" distance of P2 L31.start
  measures "d119" distance of L37.end L38.end
  measures "d120" distance of L38.end L39.end
  measures "d121" distance of L38.end L41.end
  measures "d122" distance of L43.start L43.end
  measures "d123" distance of L43.start L45.end
extrude "Extrude25" cut sketch "mounting-screws" against normal blind 24 contours A16 | A17 | A18 | A19 | A20 | A21 bodies 3
extrude "Extrude10" add sketch "electronics" along normal blind 5 contours L6 L15 L16 L17 L32 L48 L52 L53 L54 | L15 L32 L48 L52 L61 L62 | L15 L31 L32 L34 L35 L36 L40 L59 L60 L61 | L17 L18 L33 L48 L49 L51 L54 L57 L58 | L15 L28 L48 L61 L62 | L15 L25 L26 L27 L40 L59 L60 L61 | L10 L11 L12 L32 L48 L52 L53 L54 | L10 L32 L33 L48 L52 | L18 L33 L49 L50 L55 L58 | L9 L33 L48 L51 L54 | L15 L25 L26 L27 L28 L41 L47 | L9 L10 L11 L12 L33 L48 | L18 L33 L48 L51 L52 L56 L57 L62 | L33 L48 L51 L52 | L18 L33 L44 L45 L55 L58 | L18 L33 L43 L57 L58 | L15 L18 L28 L47 L48 L62 | L18 L33 L43 L44 L45 L46 | L18 L33 L50 L55 L56 L62 | L33 L34 L42 L50 L59 L62 | L18 L28 L47 L50 L62 | L34 L39 L40 L42 L59 | L25 L40 L41 L42 L59 | L18 L33 L46 L55 L56 | L18 L33 L56 L57 | L25 L28 L42 L50 L59 L62 | A8 A9 | A10 A11 bodies 3
extrude "Extrude11" add sketch "electronics" along normal blind 7 from surface at 5 contours L6 L15 L16 L17 L32 L48 L52 L53 L54 | L15 L32 L48 L52 L61 L62 | L15 L31 L32 L34 L35 L36 L40 L59 L60 L61 | L17 L18 L33 L48 L49 L51 L54 L57 L58 | L15 L28 L48 L61 L62 | L15 L25 L26 L27 L40 L59 L60 L61 | L10 L11 L12 L32 L48 L52 L53 L54 | L10 L32 L33 L48 L52 | L18 L33 L49 L50 L55 L58 | L9 L33 L48 L51 L54 | L18 L33 L48 L51 L52 L56 L57 L62 | L33 L48 L51 L52 | L18 L33 L44 L45 L55 L58 | L18 L33 L43 L57 L58 | L15 L18 L28 L47 L48 L62 | L18 L33 L50 L55 L56 L62 | L33 L34 L42 L50 L59 L62 | L18 L28 L47 L50 L62 | L18 L33 L46 L55 L56 | L18 L33 L56 L57 | L25 L28 L42 L50 L59 L62 bodies 3
extrude "Extrude12" cut sketch "electronics" along normal blind 7 from surface at 5 contours L15 L28 L48 L61 L62 | L15 L25 L26 L27 L40 L59 L60 L61 | L10 L11 L12 L32 L48 L52 L53 L54 | L10 L32 L33 L48 L52 | L9 L33 L48 L51 L54 | L33 L48 L51 L52 | L18 L33 L44 L45 L55 L58 | L18 L33 L43 L57 L58 | L15 L18 L28 L47 L48 L62 | L18 L28 L47 L50 L62 | L25 L40 L41 L42 L59 | L18 L33 L46 L55 L56 | L18 L33 L56 L57 | L25 L28 L42 L50 L59 L62 bodies 3
extrude "Extrude13" add 1 faces at (41.4583, -29.6667, -13) along direction (0.707107, -0.707107, 0) blind 0.24 on bodies 3 bodies 3
extrude "Extrude14" add 1 faces at (41.7917, 29.3333, -13) along direction (0.707107, 0.707107, 0) blind 0.24 on bodies 3 bodies 3
extrude "Extrude15" cut sketch "electronics" along normal blind 5 and the other way blind 3 contours A8 A9 | A10 A11 bodies 3
sketch "top-wire-hole-left" plane through (-37.5, -37.5, 0) normal (-0.707107, -0.707107, 0) x (0.707107, -0.707107, 0)
  line L0 (-2.0711, 0) -> (-19.1421, 0)
  line L1 (-19.1421, 0) -> (-19.1421, -24)
  line L2 (-19.1421, -24) -> (-2.0711, -24)
  line L3 (-2.0711, -24) -> (-2.0711, 0)
  line L4 (-19.1421, 0) -> (-2.0711, -24) construction
  line L5 (-2.0711, 0) -> (-19.1421, -24) construction
  circle A0 centre (-10.6066, -12) radius 4
  dimension "d144" = 8
  constraint coincident L0.end L1.start
  constraint coincident L2.end L3.start
  constraint coincident L0.start L3.end
  constraint coincident L1.end L2.start
  constraint midpoint L4 A0.centre
  measures "d144" diameter of A0
extrude "Extrude16" cut sketch "top-wire-hole-left" against normal blind 3 contours A0 bodies 3
sketch "top-wire-hole-right" plane through (-37.5, 37.5, 0) normal (-0.707107, 0.707107, 0) x (-0.707107, -0.707107, 0)
  line L0 (19.1421, 0) -> (2.0711, 0)
  line L1 (2.0711, 0) -> (2.0711, -24)
  line L2 (2.0711, -24) -> (19.1421, -24)
  line L3 (19.1421, -24) -> (19.1421, 0)
  line L4 (2.0711, 0) -> (19.1421, -24) construction
  line L5 (19.1421, 0) -> (2.0711, -24) construction
  circle A0 centre (10.6075, -12.0059) radius 4
  point P0 (10.6075, -12.0059)
  dimension "d147" = 8
  constraint coincident L0.end L1.start
  constraint coincident L2.end L3.start
  constraint coincident L0.start L3.end
  constraint coincident L1.end L2.start
  constraint coincident P0 A0.centre
  measures "d147" diameter of A0
extrude "Extrude17" cut sketch "top-wire-hole-right" against normal blind 3 contours A0 bodies 3
sketch "usb-passthrough" plane through (0, 37.5, 0) normal (0, 1, 0) x (-1, 0, 0)
  line L0 (35.4289, 0) -> (-35.4289, 0)
  line L1 (-35.4289, 0) -> (-35.4289, -24)
  line L2 (-35.4289, -24) -> (35.4289, -24)
  line L3 (35.4289, -24) -> (35.4289, 0)
  line L4 (-31.675, -9) -> (-20.675, -16) construction
  line L5 (-40.425, -16) -> (-11.925, -16) construction
  line L6 (-20.675, -16) -> (-20.675, -9) construction
  line L7 (-20.675, -9) -> (-31.675, -16) construction
  line L8 (-21.175, -7.5) -> (-31.175, -7.5) construction
  line L9 (-34.175, -10.5) -> (-34.175, -17.5)
  line L10 (-34.175, -17.5) -> (-18.175, -17.5) construction
  line L11 (-18.175, -17.5) -> (-18.175, -10.5) construction
  line L12 (-18.175, -7.5) -> (-34.175, -17.5) construction
  line L13 (-34.175, -7.5) -> (-18.175, -17.5) construction
  arc A0 (-31.175, -7.5) -> (-34.175, -10.5) centre (-31.175, -10.5) ccw construction
  arc A1 (-18.175, -10.5) -> (-21.175, -7.5) centre (-21.175, -10.5) ccw construction
  line L14 (-31.175, -7.5) -> (-31.175, -17.5) construction
  line L15 (-26.175, -12.5) -> (-26.175, -7.5) construction
  line L16 (-26.175, -12.5) -> (-26.175, -16) construction
  line L17 (-31.175, -7.5) -> (-26.175, -16) construction
  line L18 (-26.175, -7.5) -> (-31.175, -16) construction
  line L19 (-28.675, -11.75) -> (-28.675, -7.5) construction
  line L20 (-28.675, -7.5) -> (-8.675, -7.5)
  line L21 (-8.675, -7.5) -> (-8.675, -16)
  line L22 (-8.675, -16) -> (-28.675, -16)
  line L23 (-28.675, -16) -> (-28.675, -7.5)
  line L24 (-28.675, -7.5) -> (-8.675, -7.5)
  line L25 (-8.675, -7.5) -> (-8.675, -2.5)
  line L26 (-8.675, -2.5) -> (-28.675, -2.5)
  line L27 (-28.675, -2.5) -> (-28.675, -7.5)
  point P0 (-31.675, -9)
  point P1 (-20.675, -16)
  point P2 (-20.675, -9)
  point P3 (-31.675, -16)
  point P4 (-26.175, -12.5)
  dimension "d150" = 16
  dimension "d151" = 10
  dimension "d152" = 3
  dimension "d153" = 3
  dimension "d179" = 20
  dimension "d180" = 20
  dimension "d181" = 5
  constraint coincident P0 L4.start
  constraint coincident P1 L4.end
  constraint coincident P2 L6.end
  constraint coincident P3 L7.end
  constraint horizontal L8
  constraint perpendicular L8 L9
  constraint parallel L8 L10
  constraint parallel L9 L11
  constraint coincident L12 P4
  constraint coincident L13 P4
  constraint midpoint L7 P4
  constraint coincident L13.start L8
  constraint coincident L13.start L9
  constraint tangent L8 A0
  constraint tangent L9 A0
  constraint coincident L12.start L11
  constraint coincident L12.start L8
  constraint tangent L11 A1
  constraint tangent L8 A1
  constraint coincident L10 L14.end
  constraint perpendicular L10 L14
  constraint coincident P4 L15.start
  constraint midpoint L8 L15.end
  constraint midpoint L5 L16.end
  constraint coincident L14 L18.end
  constraint midpoint L17 L19.start
  constraint coincident L8 L19.end
  constraint perpendicular L8 L19
  constraint horizontal L20
  constraint vertical L21
  constraint horizontal L22
  constraint vertical L23
  constraint horizontal L24
  constraint vertical L25
  constraint horizontal L26
  constraint vertical L27
  measures "d150" distance of L9.end L10.end
  measures "d151" distance of L13.start L9.end
  measures "d152" radius of A0
  measures "d153" radius of A1
  measures "d179" distance of L19.end L20.end
  measures "d180" distance of L19.end L20.end
  measures "d181" distance of L19.end L26.end
extrude "Extrude24" cut sketch "usb-passthrough" against normal blind 2.5 contours L20 L24 L25 L26 L27 | L20 L21 L22 L23 L24 bodies 3
chamfer "Chamfer1" distance 3 angle 45 4 edges at (8.675, 36.25, -2.5) (28.675, 36.25, -16) (8.675, 36.25, -16) (28.675, 36.25, -2.5) on bodies 3
extrude "Extrude19" cut 1 faces at (-51.6667, -0.8165, 0) along direction (0, 0, -1) blind 1.5 on bodies 3 bodies 3
extrude "Extrude20" cut 1 faces at (-11.6583, -10, -9) along direction (0, 0, -1) blind 12 on bodies 3 bodies 3
extrude "Extrude21" cut 3 faces at (28.0083, -9.4333, -16) (-3.5083, 7.3667, -16) (2.2533, -20.9317, -16) along direction (0, 0, -1) blind 5 on bodies 3 bodies 3
extrude "Extrude22" add sketch "electronics" against normal blind 3 contours A8 A9 | A10 A11 bodies 3
sketch "revert" plane through (0, 0, -21) normal (0, 0, 1) x (-1, 0, 0)
  line L0 (35.4289, 35) -> (-35.4289, 35)
  arc A0 (-35.4289, 35) -> (-37.1967, 34.2678) centre (-35.4289, 32.5) ccw
  line L1 (-37.1967, 34.2678) -> (-49.2678, 22.1967)
  arc A1 (-49.2678, 22.1967) -> (-50, 20.4289) centre (-47.5, 20.4289) ccw
  line L2 (-50, 20.4289) -> (-50, -20.4289)
  arc A2 (-50, -20.4289) -> (-49.2678, -22.1967) centre (-47.5, -20.4289) ccw
  line L3 (-49.2678, -22.1967) -> (-37.1967, -34.2678)
  arc A3 (-37.1967, -34.2678) -> (-35.4289, -35) centre (-35.4289, -32.5) ccw
  line L4 (-35.4289, -35) -> (35.4289, -35)
  arc A4 (35.4289, -35) -> (37.1967, -34.2678) centre (35.4289, -32.5) ccw
  line L5 (37.1967, -34.2678) -> (49.2678, -22.1967)
  arc A5 (49.2678, -22.1967) -> (50, -20.4289) centre (47.5, -20.4289) ccw
  line L6 (50, -20.4289) -> (50, 20.4289)
  arc A6 (50, 20.4289) -> (49.2678, 22.1967) centre (47.5, 20.4289) ccw
  line L7 (49.2678, 22.1967) -> (37.1967, 34.2678)
  arc A7 (37.1967, 34.2678) -> (35.4289, 35) centre (35.4289, 32.5) ccw
  line L8 (-35.4289, 35) -> (-35.4289, -35) construction
  line L9 (-35.4289, 35) -> (-34.4289, 35) construction
  line L10 (-34.4289, 35) -> (-34.4289, 32.75) construction
  line L11 (-34.4289, 32.75) -> (-6.4289, 32.75) construction
  line L12 (-6.4289, 32.75) -> (-6.4289, -32.25) construction
  line L13 (-6.4289, -32.25) -> (-34.4289, -32.25) construction
  line L14 (-34.4289, -32.25) -> (-34.4289, 32.75) construction
  line L15 (-34.4289, 32.75) -> (-6.4289, -32.25) construction
  line L16 (-6.4289, 32.75) -> (-34.4289, -32.25) construction
  circle A8 centre (-20.4289, 0.25) radius 1.6
  line L17 (-20.4289, 32.75) -> (-20.4289, -32.25) construction
  line L18 (-34.4289, 0.25) -> (-6.4289, 0.25) construction
  line L19 (-34.4289, 32.75) -> (-6.4289, 0.25) construction
  line L20 (-6.4289, 32.75) -> (-34.4289, 0.25) construction
  circle A9 centre (-20.4289, 16.5) radius 1.6
  line L21 (-34.4289, -32.25) -> (-6.4289, 0.25) construction
  line L22 (-34.4289, 0.25) -> (-6.4289, -32.25) construction
  circle A10 centre (-20.4289, -16) radius 1.6
  circle A11 centre (0, 0) radius 1.6
  circle A12 centre (18, 0) radius 1.6
  line L23 (-20.4289, 16.5) -> (18, 16.5) construction
  line L24 (0, 16.5) -> (0, -16) construction
  line L25 (-20.4289, -16) -> (18, -16) construction
  circle A13 centre (0, -16) radius 1.6
  circle A14 centre (18, -16) radius 1.6
  circle A15 centre (18, 16.5) radius 1.6
  circle A16 centre (0, 16.5) radius 1.6
  circle A17 centre (47.5, -10.2145) radius 1.55
  circle A18 centre (-47.5, 10.2145) radius 1.55
  circle A19 centre (47.5, -0.0001) radius 1.55
  circle A20 centre (-47.5, -10.2145) radius 1.55
  circle A21 centre (-47.5, 0) radius 1.55
  circle A22 centre (47.5, 10.2145) radius 1.55
  point P0 (-35.4289, 35)
  dimension "d164" = 1
  dimension "d165" = 2.25
  dimension "d166" = 28
  dimension "d167" = 65
  dimension "d168" = 3.2
  dimension "d169" = 3.2
  dimension "d170" = 3.2
  dimension "d171" = 3.2
  dimension "d172" = 3.2
  dimension "d173" = 3.2
  dimension "d174" = 3.2
  dimension "d175" = 3.2
  dimension "d176" = 3.2
  constraint coincident P0 L0.end
  constraint coincident A3.end L4.start
  constraint parallel L0 L9
  constraint perpendicular L9 L10
  constraint horizontal L11
  constraint vertical L12
  constraint horizontal L13
  constraint vertical L14
  constraint midpoint L15 A8.centre
  constraint midpoint L11 L17.start
  constraint midpoint L13 L17.end
  constraint midpoint L14 L18.start
  constraint midpoint L12 L18.end
  constraint midpoint L19 A9.centre
  constraint midpoint L22 A10.centre
  constraint coincident A11.centre origin
  constraint coincident A9.centre L23.start
  constraint horizontal L23
  constraint coincident L23 L24.start
  constraint perpendicular L23 L24
  constraint coincident A10.centre L25.start
  constraint horizontal L25
  constraint coincident L24.end A13.centre
  constraint coincident L25.end A14.centre
  constraint coincident L23.end A15.centre
  constraint coincident L24.start A16.centre
  measures "d164" distance of P0 L9.end
  measures "d165" distance of L9.end L10.end
  measures "d166" distance of L10.end L11.end
  measures "d167" distance of L10.end L13.end
  measures "d168" diameter of A8
  measures "d169" diameter of A9
  measures "d170" diameter of A10
  measures "d171" diameter of A11
  measures "d172" diameter of A12
  measures "d173" diameter of A13
  measures "d174" diameter of A14
  measures "d175" diameter of A15
  measures "d176" diameter of A16
extrude "Extrude23" cut sketch "revert" against normal blind 3 contours A8 | A9 | A10 | A11 | A12 | A13 | A14 | A15 | A16 bodies 3
equation "d4 = 68 mm + 1 mm"
equation "d13 = 34 mm + 0.6 mm"
equation "d14 = 34 mm + 0.6 mm"
equation "d44 = d43"
equation "d46 = d45"
equation "d48 = d47"
equation "d50 = d49"
equation "d107 = 2 mm + ( ( 15.8 / 2 ) * 1 mm )"
equation "d116 = d115"
equation "d118 = d117"
equation "d133 = 12 mm - 5 mm"
named bodies: "load-cell-bracket", "load-cell-lid", "circuit-box"
